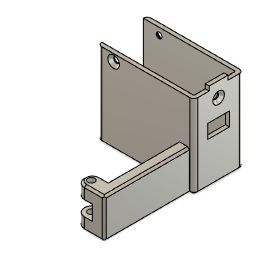
N4M Webcam Mount X (Autodesk Fusion 360 design; units mm, degrees)
Autodesk Fusion 360 part; units mm, degrees
sketch "Skizze1" plane through (0, 0, 0) normal (0, 1, 0) x (1, 0, 0)
  line L0 (-24.25, 12.5) -> (24.25, 12.5)
  line L1 (24.25, 12.5) -> (24.25, -12.5)
  line L2 (24.25, -12.5) -> (-24.25, -12.5)
  line L3 (-24.25, -12.5) -> (-24.25, 12.5)
  line L4 (-24.25, 12.5) -> (24.25, -12.5) construction
  line L5 (24.25, 12.5) -> (-24.25, -12.5) construction
  line L6 (22.25, -10.5) -> (-22.25, -10.5)
  line L7 (-22.25, -10.5) -> (-22.25, 10.5)
  line L8 (-22.25, 10.5) -> (22.25, 10.5)
  line L9 (22.25, 10.5) -> (22.25, -10.5)
  line L10 (-22.25, -10.5) -> (-24.25, -10.5)
  line L11 (-22.25, 10.5) -> (-24.25, 10.5)
  dimension "d1" = 48.5
  dimension "d2" = 25
  dimension "d3" = 2
  constraint horizontal L0
  constraint perpendicular L0 L1
  constraint parallel L0 L2
  constraint parallel L1 L3
  constraint coincident L4 origin
  constraint coincident L5 origin
  constraint coincident L3 L10.end
  constraint perpendicular L3 L10
  constraint coincident L3 L11.end
  constraint perpendicular L3 L11
  measures "d1" distance of L1.end L2.end
  measures "d2" distance of L0.end L1.end
extrude "Extrusion1" add sketch "Skizze1" along normal blind 2 contours L6 L7 L8 L9
extrude "Extrusion3" add sketch "Skizze1" along normal blind 42 contours L0 L1 L2 L3 L6 L8 L9 L10 L11
sketch "Skizze2" plane through (0, 0, 12.5) normal (0, 0, 1) x (1, 0, 0)
  line L0 (-24.25, 0) -> (24.25, 0)
  line L1 (24.25, 0) -> (24.25, 42)
  line L2 (24.25, 42) -> (-24.25, 42)
  line L3 (-24.25, 42) -> (-24.25, 0)
  circle A0 centre (-16.25, 38.4702) radius 1.45
  dimension "d11" = 2.9
  measures "d11" diameter of A0
sketch "Skizze3" plane through (0, 0, -12.5) normal (0, 0, -1) x (-1, 0, 0)
  line L0 (-24.25, 0) -> (24.25, 0)
  line L1 (24.25, 0) -> (24.25, 42)
  line L2 (24.25, 42) -> (-24.25, 42)
  line L3 (-24.25, 42) -> (-24.25, 0)
  circle A0 centre (16.25, 38.4702) radius 1.45
  dimension "d12" = 2.9
  measures "d12" diameter of A0
extrude "Extrusion4" cut sketch "Skizze3" against normal blind 2 contours A0
extrude "Extrusion5" cut sketch "Skizze2" against normal blind 2 contours A0
chamfer "Fase1" distance 1.5 angle 45 1 edges at (-17.6019, 38.9946, 12.5)
chamfer "Fase2" distance 1.5 angle 45 1 edges at (-14.8981, 38.9946, -12.5)
sketch "Skizze4" plane through (0, 42, 0) normal (0, 1, 0) x (-1, 0, 0)
  line L0 (-22.25, -10.5) -> (-22.25, 10.5)
  line L1 (-22.25, 10.5) -> (24.25, 10.5)
  line L2 (24.25, 10.5) -> (24.25, 12.5)
  line L3 (24.25, 12.5) -> (-24.25, 12.5)
  line L4 (-24.25, 12.5) -> (-24.25, -12.5)
  line L5 (-24.25, -12.5) -> (24.25, -12.5)
  line L6 (24.25, -12.5) -> (24.25, -10.5)
  line L7 (24.25, -10.5) -> (-22.25, -10.5)
  line L8 (-22.25, -4.75) -> (-24.25, -4.75)
  line L9 (-24.25, -4.75) -> (-24.25, 4.75)
  line L10 (-24.25, 4.75) -> (-22.25, 4.75)
  line L11 (-22.25, 4.75) -> (-22.25, -4.75)
  line L12 (-22.25, -4.75) -> (-24.25, 4.75) construction
  line L13 (-24.25, -4.75) -> (-22.25, 4.75) construction
  point P0 (-23.25, 0)
  dimension "d20" = 2
  dimension "d21" = 9.5
  constraint horizontal L8
  constraint perpendicular L8 L9
  constraint parallel L8 L10
  constraint parallel L9 L11
  constraint coincident L12 P0
  constraint coincident L13 P0
  measures "d20" distance of L9.end L10.end
  measures "d21" distance of L8.end L9.end
extrude "Extrusion6" add sketch "Skizze4" along normal blind 2.2 contours L0 L4 L8 L9 L10 L11
sketch "Skizze5" plane through (24.25, 0, 0) normal (1, 0, 0) x (0, 0, -1)
  line L0 (-12.5, 0) -> (12.5, 0)
  line L1 (12.5, 0) -> (12.5, 42)
  line L2 (12.5, 42) -> (4.75, 42)
  line L3 (4.75, 42) -> (4.75, 44.2)
  line L4 (4.75, 44.2) -> (-4.75, 44.2)
  line L5 (-4.75, 44.2) -> (-4.75, 42)
  line L6 (-4.75, 42) -> (-12.5, 42)
  line L7 (-12.5, 42) -> (-12.5, 0)
  circle A0 centre (0, 36.7) radius 1.45
  line L8 (5.5, 21.2) -> (-5.5, 21.2)
  line L9 (-5.5, 21.2) -> (-5.5, 28.2)
  line L10 (-5.5, 28.2) -> (5.5, 28.2)
  line L11 (5.5, 28.2) -> (5.5, 21.2)
  line L12 (5.5, 21.2) -> (-5.5, 28.2) construction
  line L13 (-5.5, 21.2) -> (5.5, 28.2) construction
  point P0 (0, 24.7)
  dimension "d25" = 2.9
  dimension "d27" = 11
  dimension "d28" = 7
  constraint horizontal L8
  constraint perpendicular L8 L9
  constraint parallel L8 L10
  constraint parallel L9 L11
  constraint coincident L12 P0
  constraint coincident L13 P0
  measures "d25" diameter of A0
  measures "d27" distance of L9.end L10.end
  measures "d28" distance of L8.end L9.end
extrude "Extrusion7" cut sketch "Skizze5" against normal blind 2 contours A0 | L8 L9 L10 L11
chamfer "Fase3" distance 1.5 angle 45 1 edges at (24.25, 37.2243, 1.3519)
extrude "Extrusion8" add sketch "Skizze1" along normal blind 2 contours L3 L7 L10 L11
sketch "Skizze6" plane through (0, 2, 0) normal (0, 1, 0) x (-1, 0, 0)
  line L0 (-22.25, -10.5) -> (24.25, -10.5)
  line L1 (24.25, -10.5) -> (24.25, 10.5)
  line L2 (24.25, 10.5) -> (-22.25, 10.5)
  line L3 (-22.25, 10.5) -> (-22.25, -10.5)
  line L4 (11.15, -10.5) -> (10.35, -10.5)
  line L5 (10.35, -10.5) -> (10.35, 10.5)
  line L6 (10.35, 10.5) -> (11.15, 10.5)
  line L7 (11.15, 10.5) -> (11.15, -10.5)
  line L8 (11.15, -10.5) -> (10.35, 10.5) construction
  line L9 (10.35, -10.5) -> (11.15, 10.5) construction
  line L10 (-6.85, -10.5) -> (-7.65, -10.5)
  line L11 (-7.65, -10.5) -> (-7.65, 10.5)
  line L12 (-7.65, 10.5) -> (-6.85, 10.5)
  line L13 (-6.85, 10.5) -> (-6.85, -10.5)
  line L14 (-6.85, -10.5) -> (-7.65, 10.5) construction
  line L15 (-7.65, -10.5) -> (-6.85, 10.5) construction
  line L16 (-7.65, 10.5) -> (-6.85, 10.5)
  line L17 (-6.85, 10.5) -> (-6.85, 8)
  line L18 (-6.85, 8) -> (-7.65, 8)
  line L19 (-7.65, 8) -> (-7.65, 10.5)
  line L20 (10.35, 10.5) -> (11.15, 10.5)
  line L21 (11.15, 10.5) -> (11.15, 8)
  line L22 (11.15, 8) -> (10.35, 8)
  line L23 (10.35, 8) -> (10.35, 10.5)
  line L24 (-7.65, -10.5) -> (-6.85, -10.5)
  line L25 (-6.85, -10.5) -> (-6.85, -8)
  line L26 (-6.85, -8) -> (-7.65, -8)
  line L27 (-7.65, -8) -> (-7.65, -10.5)
  line L28 (10.35, -10.5) -> (11.15, -10.5)
  line L29 (11.15, -10.5) -> (11.15, -8)
  line L30 (11.15, -8) -> (10.35, -8)
  line L31 (10.35, -8) -> (10.35, -10.5)
  line L32 (-6.85, 0.4172) -> (10.35, 0.4172)
  line L33 (10.35, 0.4172) -> (10.35, -0.3828)
  line L34 (10.35, -0.3828) -> (-6.85, -0.3828)
  line L35 (-6.85, -0.3828) -> (-6.85, 0.4172)
  line L36 (24.25, 10.5) -> (22.25, 10.5)
  line L37 (22.25, 10.5) -> (22.25, -10.5)
  line L38 (22.25, -10.5) -> (24.25, -10.5)
  line L39 (24.25, -10.5) -> (24.25, 10.5)
  point P0 (10.75, 0)
  point P1 (-7.25, 0)
  dimension "d35" = 18
  dimension "d36" = 0.8
  dimension "d37" = 21
  dimension "d38" = 0.8
  dimension "d39" = 21
  dimension "d40" = 0.8
  dimension "d41" = 2.5
  dimension "d42" = 2.5
  dimension "d43" = 2.5
  dimension "d44" = 2.5
  dimension "d49" = 0.8
  dimension "d50" = 2
  constraint horizontal L4
  constraint perpendicular L4 L5
  constraint parallel L4 L6
  constraint parallel L5 L7
  constraint coincident L8 P0
  constraint coincident L9 P0
  constraint horizontal L10
  constraint perpendicular L10 L11
  constraint parallel L10 L12
  constraint parallel L11 L13
  constraint coincident L14 P1
  constraint coincident L15 P1
  constraint horizontal L16
  constraint vertical L17
  constraint horizontal L18
  constraint vertical L19
  constraint horizontal L20
  constraint vertical L21
  constraint horizontal L22
  constraint vertical L23
  constraint horizontal L24
  constraint vertical L25
  constraint horizontal L26
  constraint vertical L27
  constraint horizontal L28
  constraint vertical L29
  constraint horizontal L30
  constraint vertical L31
  constraint horizontal L32
  constraint vertical L33
  constraint horizontal L34
  constraint vertical L35
  constraint coincident L13 L32.start
  constraint horizontal L36
  constraint vertical L37
  constraint horizontal L38
  constraint vertical L39
  constraint coincident L1.end L2.start
  measures "d35" distance of P0 P1
  measures "d36" distance of L5.end L6.end
  measures "d37" distance of L4.end L5.end
  measures "d38" distance of L11.end L12.end
  measures "d39" distance of L10.end L11.end
  measures "d40" distance of L11.end L12.end
  measures "d41" distance of L11.end L18.end
  measures "d42" distance of L5.end L22.end
  measures "d43" distance of L10.end L26.end
  measures "d44" distance of L4.end L30.end
  measures "d49" distance of L32.start L34.end
  measures "d50" distance of L1.end L36.end
extrude "Extrusion9" add sketch "Skizze6" along normal blind 10 contours L11 L13 L18 L26 L35 | L5 L7 L22 L30 L33
extrude "Extrusion10" add sketch "Skizze6" along normal blind 19 contours L0 L10 L11 L13 L24 L25 L26 L27 | L2 L11 L12 L13 L16 L17 L18 L19 | L0 L4 L5 L7 L28 L29 L30 L31 | L2 L5 L6 L7 L20 L21 L22 L23
extrude "Extrusion12" add sketch "Skizze6" along normal blind 19 contours L0 L1 L2 L36 L37 L38 L39
extrude "Extrusion13" add sketch "Skizze6" along normal blind 8 contours L5 L13 L32 L33 L34 L35
chamfer "Fase4" distance 1 angle 45 4 edges at (-10.75, 21, 8) (7.25, 21, 8) (-10.75, 21, -8) (7.25, 21, -8)
fillet "Abrundung1" radius 2 2 edges at (24.25, 21, -12.5) (24.25, 21, 12.5)
fillet "Abrundung2" radius 0.5 2 edges at (22.25, 22, 10.5) (22.25, 22, -10.5)
fillet "Abrundung3" radius 2 2 edges at (-24.25, 21, 12.5) (-24.25, 21, -12.5)
sketch "Skizze8" plane through (0, 0, 12.5) normal (0, 0, 1) x (1, 0, 0)
  line L0 (-22.25, 42) -> (-22.25, 0)
  line L1 (-22.25, 0) -> (22.25, 0)
  line L2 (22.25, 0) -> (22.25, 42)
  line L3 (22.25, 42) -> (-22.25, 42)
  circle A0 centre (-16.25, 38.4702) radius 2.95
  line L4 (22, 0) -> (16, 0)
  line L5 (16, 0) -> (16, 20)
  line L6 (16, 20) -> (22, 20)
  line L7 (22, 20) -> (22, 0)
  line L8 (22, 0) -> (16, 20) construction
  line L9 (16, 0) -> (22, 20) construction
  point P0 (19, 10)
  dimension "d68" = 6
  dimension "d69" = 20
  constraint horizontal L4
  constraint perpendicular L4 L5
  constraint parallel L4 L6
  constraint parallel L5 L7
  constraint coincident L8 P0
  constraint coincident L9 P0
  measures "d68" distance of L5.end L6.end
  measures "d69" distance of L4.end L5.end
extrude "Extrusion15" add sketch "Skizze8" along normal blind 43 contours L1 L4 L5 L6 L7
sketch "Skizze9" plane through (16, 0, 0) normal (-1, 0, 0) x (0, 0, 1)
  line L0 (12.5, 20) -> (12.5, 0)
  line L1 (12.5, 0) -> (55.5, 0)
  line L2 (55.5, 0) -> (55.5, 20)
  line L3 (55.5, 20) -> (12.5, 20)
  line L4 (55.5, 20) -> (47.5, 20)
  line L5 (47.5, 20) -> (47.5, 0)
  line L6 (47.5, 0) -> (55.5, 0)
  line L7 (55.5, 0) -> (55.5, 20)
  dimension "d72" = 8
  constraint horizontal L4
  constraint vertical L5
  constraint horizontal L6
  constraint vertical L7
  constraint coincident L2.end L3.start
  measures "d72" distance of L2.end L4.end
extrude "Extrusion16" add sketch "Skizze9" along normal blind 8 contours L1 L2 L3 L4 L5 L6 L7
sketch "Skizze10" plane through (0, 0, 0) normal (0, -1, 0) x (1, 0, 0)
  line L0 (8, 47.5) -> (16, 47.5)
  line L1 (16, 47.5) -> (16, 12.5)
  line L2 (22.25, 12.5) -> (22, 12.5)
  arc A0 (-22.25, 12.5) -> (-24.25, 10.5) centre (-22.25, 10.5) ccw
  line L3 (-24.25, 10.5) -> (-24.25, -10.5)
  arc A1 (-24.25, -10.5) -> (-22.25, -12.5) centre (-22.25, -10.5) ccw
  line L4 (-22.25, -12.5) -> (22.25, -12.5)
  arc A2 (22.25, -12.5) -> (24.25, -10.5) centre (22.25, -10.5) ccw
  line L5 (24.25, -10.5) -> (24.25, 10.5)
  arc A3 (24.25, 10.5) -> (22.25, 12.5) centre (22.25, 10.5) ccw
  line L6 (22, 12.5) -> (22, 55.5)
  line L7 (22, 55.5) -> (8, 55.5)
  circle A4 centre (11.5, 51.5) radius 1.75
  line L8 (8, 55.5) -> (8, 47.5)
  line L9 (16, 12.5) -> (-22.25, 12.5)
  dimension "d77" = 3.5
  measures "d77" diameter of A4
extrude "Extrusion17" cut sketch "Skizze10" against normal blind 20 contours A4
sketch "Skizze11" plane through (8, 0, 0) normal (-1, 0, 0) x (0, 0, 1)
  line L0 (55.5, 0) -> (55.5, 20)
  line L1 (55.5, 20) -> (47.5, 20)
  line L2 (47.5, 20) -> (47.5, 0)
  line L3 (47.5, 0) -> (55.5, 0)
  line L4 (55.5, 6.25) -> (47.5, 6.25)
  line L5 (47.5, 6.25) -> (47.5, 13.75)
  line L6 (47.5, 13.75) -> (55.5, 13.75)
  line L7 (55.5, 13.75) -> (55.5, 6.25)
  line L8 (55.5, 6.25) -> (47.5, 13.75) construction
  line L9 (47.5, 6.25) -> (55.5, 13.75) construction
  point P0 (51.5, 10)
  dimension "d80" = 7.5
  constraint horizontal L4
  constraint perpendicular L4 L5
  constraint parallel L4 L6
  constraint parallel L5 L7
  constraint coincident L8 P0
  constraint coincident L9 P0
  measures "d80" distance of L4.end L5.end
extrude "Extrusion18" cut sketch "Skizze11" against normal blind 8 contours L0 L2 L4 L5 L6 L7
fillet "Abrundung5" radius 4 4 edges at (8, 16.875, 47.5) (8, 16.875, 55.5) (8, 3.125, 47.5) (8, 3.125, 55.5)
chamfer "Fase10" distance 1 angle 45 19 edges at (14, 0, 47.5) (8, 0, 51.5) (17, 0, 55.5) (22, 0, 34) (23.6642, 0, 11.9142) (24.25, 0, 0) (23.6642, 0, -11.9142) (0, 0, -12.5) (-23.6642, 0, -11.9142) (-24.25, 0, 0) (-23.6642, 0, 11.9142) (-3.125, 0, 12.5) (22.125, 0, 12.5) (16, 0, 30) (22, 20, 34) (17, 20, 55.5) (8, 20, 51.5) (14, 20, 47.5) (16, 20, 30)
chamfer "Fase11" distance 1 angle 45 1 edges at (22, 10, 55.5)
